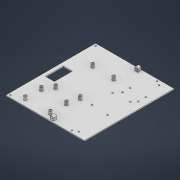
# Autodesk Inventor part: Obenplatte_vorne
Saved by Autodesk Inventor 2021 (Build 250183000, 183)
## iProperties
Created: 2021-02-01
Part Number: Obenplatte_vorne
Material: Generisch
Document SubType Name: Modeling
Designer: laure
Density: 1 g/cm^3
Appearance: Vorgabe
Author: laure
Autodesk Inventor part; units mm, degrees
ref_plane "YZ Plane" through (0, 0, 0) normal (1, 0, 0) x (0, 1, 0)
ref_plane "XZ Plane" through (0, 0, 0) normal (0, 1, 0) x (-1, 0, 0)
ref_plane "XY Plane" through (0, 0, 0) normal (0, 0, 1) x (1, 0, 0)
sketch "Skizze1" plane through (0, 0, 0) normal (0, 1, 0) x (-1, 0, 0)
  line L0 (87.5, -100) -> (-87.5, -100)
  line L1 (-87.5, -100) -> (-87.5, 100)
  line L2 (-87.5, 100) -> (87.5, 100)
  line L3 (87.5, 100) -> (87.5, -100)
  line L4 (0, -140) -> (0, 140) projected
  line L5 (122.5, 0) -> (-122.5, 0) projected
  point P0 (0, 0)
  dimension "d0" = 175
  dimension "d1" = 200
  constraints: 8 end point, 2 parallel, 1 horizontal, 1 perpendicular, 2 other
  measures "d0" distance of L1.end L2.end
  measures "d1" distance of L0.end L1.end
extrude "Extrusion1" add sketch "Skizze1" along normal blind 2
sketch "Skizze2" plane through (0, 2, 0) normal (0, 1, 0) x (1, 0, 0)
  circle A0 centre (54.5, 95) radius 1.6
  circle A1 centre (-82.5, 95) radius 1.6
  line L0 (0, 140) -> (0, -140) projected
  line L1 (122.5, 0) -> (-122.5, 0) projected
  line L2 (87.5, 100) -> (-87.5, 100) projected
  circle A2 centre (54.5, -95) radius 1.6
  circle A3 centre (-82.5, -95) radius 1.6
  line L3 (-87.5, 100) -> (-87.5, -100) projected
  line L4 (87.5, -100) -> (87.5, 100) projected
  point P0 (0, 0)
  dimension "d4" = 3.2
  dimension "d5" = 3.2
  dimension "d7" = 5
  dimension "d9" = 5
  dimension "d55" = 5
  dimension "d56" = 33
  constraints: 4 centre point, 2 symmetric about line, 2 other
  measures "d4" diameter of A0
  measures "d5" diameter of A1
  measures "d7" distance from line of L2 A0.centre
  measures "d9" distance from line of L2 A1.centre
  measures "d55" distance from line of L3 A1.centre
  measures "d56" distance from line of L4 A0.centre
extrude "Extrusion2" cut sketch "Skizze2" against normal up to surface (2 mm away) contours A0 | A1 | A2 | A3
sketch "Skizze3" plane through (0, 2, 0) normal (0, 1, 0) x (1, 0, 0)
  line L0 (0, 140) -> (0, -140) projected
  line L1 (122.5, 0) -> (-122.5, 0) projected
  line L2 (-87.5, -100) -> (87.5, -100) projected
  line L3 (-87.5, 100) -> (-87.5, -100) projected
  circle A0 centre (64.5, -89.5) radius 1.6
  line L4 (87.5, -100) -> (87.5, 100) projected
  circle A1 centre (64.5, -25.5) radius 1.6
  circle A2 centre (64.5, 25.5) radius 1.6
  line L5 (87.5, 100) -> (-87.5, 100) projected
  circle A3 centre (64.5, 89.5) radius 1.6
  circle A4 centre (27.5, -23) radius 1.6
  circle A5 centre (27.5, 23) radius 1.6
  point P0 (0, 0)
  dimension "d35" = 3.2
  dimension "d36" = 10.5
  dimension "d37" = 23
  dimension "d38" = 3.2
  dimension "d39" = 74.5
  dimension "d40" = 23
  dimension "d41" = 3.2
  dimension "d42" = 23
  dimension "d43" = 74.5
  dimension "d44" = 3.2
  dimension "d45" = 23
  dimension "d46" = 10.5
  dimension "d47" = 3.2
  dimension "d48" = 60
  dimension "d49" = 77
  dimension "d50" = 3.2
  dimension "d51" = 60
  dimension "d52" = 77
  constraints: 6 centre point
  measures "d35" diameter of A0
  measures "d36" distance from line of L2 A0.centre
  measures "d37" distance from line of L4 A0.centre
  measures "d38" diameter of A1
  measures "d39" distance from line of L2 A1.centre
  measures "d40" distance from line of L4 A1.centre
  measures "d41" diameter of A2
  measures "d42" distance from line of L4 A2.centre
  measures "d43" distance from line of L5 A2.centre
  measures "d44" diameter of A3
  measures "d45" distance from line of L4 A3.centre
  measures "d46" distance from line of L5 A3.centre
  measures "d47" diameter of A4
  measures "d48" distance from line of L4 A4.centre
  measures "d49" distance from line of L2 A4.centre
  measures "d50" diameter of A5
  measures "d51" distance from line of L4 A5.centre
  measures "d52" distance from line of L5 A5.centre
extrude "Extrusion3" cut sketch "Skizze3" against normal up to surface (2 mm away) contours A0 | A1 | A2 | A3 | A4 | A5
sketch "Skizze4" plane through (0, 2, 0) normal (0, 1, 0) x (1, 0, 0)
  line L0 (-47.5, -36.6) -> (5.84, -36.6)
  line L1 (5.84, -36.6) -> (5.84, 65)
  line L2 (5.84, 65) -> (-47.5, 65)
  line L3 (-47.5, 65) -> (-47.5, -36.6)
  line L4 (122.5, 0) -> (-122.5, 0) projected
  line L5 (-87.5, 100) -> (-87.5, -100) projected
  circle A0 centre (3.3, 49.76) radius 3.5
  circle A1 centre (3.3, -25.17) radius 3.5
  circle A2 centre (-44.96, -31.52) radius 3.5
  circle A3 centre (-44.96, 51.03) radius 3.5
  line L6 (87.5, 100) -> (-87.5, 100) projected
  point P0 (0, 0)
  point P1 (-15.83, 0)
  dimension "d57" = 53.34
  dimension "d58" = 101.6
  dimension "d59" = 40
  dimension "d60" = 7
  dimension "d61" = 86.36
  dimension "d62" = 50.8
  dimension "d63" = 7
  dimension "d64" = 90.17
  dimension "d65" = 50.8
  dimension "d66" = 7
  dimension "d67" = 96.52
  dimension "d68" = 50.8
  dimension "d69" = 7
  dimension "d70" = 87.63
  dimension "d71" = 50.8
  dimension "d140" = 35
  constraints: 8 end point, 4 centre point, 2 parallel, 1 horizontal, 1 perpendicular
  measures "d57" distance of L2.end L1.end
  measures "d58" distance of L1.end L0.end
  measures "d59" distance between parallel lines of L5 L3
  measures "d60" diameter of A0
  measures "d61" distance from line of L0 A0.centre
  measures "d62" distance from line of L3 A0.centre
  measures "d63" diameter of A1
  measures "d64" distance from line of L2 A1.centre
  measures "d65" distance from line of L3 A1.centre
  measures "d66" diameter of A2
  measures "d67" distance from line of L2 A2.centre
  measures "d68" distance from line of L1 A2.centre
  measures "d69" diameter of A3
  measures "d70" distance from line of L0 A3.centre
  measures "d71" distance from line of L1 A3.centre
  measures "d140" distance between parallel lines of L6 L2
extrude "Extrusion4" add sketch "Skizze4" along normal blind 7 contours A2 L3 | L3 A2 | A1 L1 | L1 A1 | A3 L3 | L3 A3 | A0 L1 | L1 A0
sketch "Skizze5" plane through (3.3, 9, -49.76) normal (0, 1, 0) x (1, 0, 0)
  circle A0 centre (0, 0) radius 3.5 projected
  circle A1 centre (-48.26, 1.27) radius 3.5 projected
  circle A2 centre (-48.26, -81.28) radius 3.5 projected
  circle A3 centre (0, -74.93) radius 3.5 projected
  circle A4 centre (0, 0) radius 2
  circle A5 centre (0, -74.93) radius 2
  circle A6 centre (-48.26, 1.27) radius 2
  circle A7 centre (-48.26, -81.28) radius 2
  point P0 (-3.3, -49.76)
  dimension "d74" = 4
  dimension "d75" = 4
  dimension "d76" = 4
  dimension "d77" = 4
  constraints: 4 centre point, 4 coincident
  measures "d74" diameter of A4
  measures "d75" diameter of A5
  measures "d76" diameter of A6
  measures "d77" diameter of A7
extrude "Extrusion5" cut sketch "Skizze5" against normal blind 5 contours A4 | A5 | A6 | A7
sketch "Skizze6" plane through (0, 2, 0) normal (0, 1, 0) x (1, 0, 0)
  circle A0 centre (72.5, 35) radius 1.6
  circle A1 centre (72.5, 52) radius 1.6
  line L0 (87.5, -100) -> (87.5, 100) projected
  line L1 (-122.5, 0) -> (122.5, 0) projected
  circle A2 centre (37.5, 35) radius 1.6
  circle A3 centre (37.5, 52) radius 1.6
  point P0 (0, 0)
  dimension "d80" = 3.2
  dimension "d81" = 3.2
  dimension "d82" = 15
  dimension "d83" = 15
  dimension "d84" = 35
  dimension "d85" = 17
  dimension "d88" = 3.2
  dimension "d89" = 3.2
  dimension "d90" = 50
  dimension "d91" = 50
  dimension "d92" = 35
  dimension "d94" = 17
  constraints: 4 centre point
  measures "d80" diameter of A0
  measures "d81" diameter of A1
  measures "d82" distance from line of L0 A0.centre
  measures "d83" distance from line of L0 A1.centre
  measures "d84" distance from line of L1 A0.centre
  measures "d85" distance of A0.centre A1.centre
  measures "d88" diameter of A2
  measures "d89" diameter of A3
  measures "d90" distance from line of L0 A2.centre
  measures "d91" distance from line of L0 A3.centre
  measures "d92" distance from line of L1 A2.centre
  measures "d94" distance of A2.centre A3.centre
extrude "Extrusion6" cut sketch "Skizze6" against normal up to surface (2 mm away)
sketch "Skizze7" plane through (0, 2, 0) normal (0, 1, 0) x (1, 0, 0)
  line L0 (16, -90.8) -> (9, -90.8)
  line L1 (9, -90.8) -> (9, -97.8)
  line L2 (9, -97.8) -> (16, -97.8)
  line L3 (16, -97.8) -> (16, -90.8)
  line L4 (-87.5, 100) -> (-87.5, -100) projected
  line L5 (-87.5, -100) -> (87.5, -100) projected
  line L6 (122.5, 0) -> (-122.5, 0) projected
  line L7 (16, 90.8) -> (9, 90.8)
  line L8 (9, 90.8) -> (9, 97.8)
  line L9 (9, 97.8) -> (16, 97.8)
  line L10 (16, 97.8) -> (16, 90.8)
  point P0 (0, 0)
  dimension "d95" = 103.5
  dimension "d96" = 7
  dimension "d97" = 7
  dimension "d98" = 2.2
  constraints: 16 end point, 4 symmetric about line, 2 parallel, 1 horizontal, 1 perpendicular
  measures "d95" distance between parallel lines of L4 L3
  measures "d96" distance between parallel lines of L3 L1
  measures "d97" distance between parallel lines of L2 L0
  measures "d98" distance between parallel lines of L5 L2
extrude "Extrusion7" add sketch "Skizze7" along normal blind 9
sketch "Skizze8" plane through (9, 2, 97.8) normal (0, 0, 1) x (1, 0, 0)
  circle A0 centre (3.5, 5) radius 2
  line L0 (7, 0) -> (0, 0) projected
  line L1 (7, 0) -> (7, 9) projected
  point P0 (-9, -2)
  dimension "d101" = 4
  dimension "d102" = 5
  dimension "d103" = 3.5
  constraints: 1 centre point
  measures "d101" diameter of A0
  measures "d102" distance from line of L0 A0.centre
  measures "d103" distance from line of L1 A0.centre
extrude "Extrusion8" cut sketch "Skizze8" against normal blind 5
sketch "Skizze9" plane through (16, 2, -97.8) normal (0, 0, -1) x (-1, 0, 0)
  circle A0 centre (3.5, 5) radius 2
  line L0 (7, 0) -> (7, 9) projected
  line L1 (7, 0) -> (0, 0) projected
  point P0 (16, -2)
  dimension "d107" = 4
  dimension "d108" = 3.5
  dimension "d109" = 5
  constraints: 1 centre point
  measures "d107" diameter of A0
  measures "d108" distance from line of L0 A0.centre
  measures "d109" distance from line of L1 A0.centre
extrude "Extrusion9" cut sketch "Skizze9" against normal blind 5
fillet "Rundung1" radius 3.5 4 edges at (16, 11, -94.3) (9, 11, -94.3) (9, 11, 94.3) (16, 11, 94.3)
sketch "Skizze10" plane through (0, 2, 0) normal (0, 1, 0) x (1, 0, 0)
  line L0 (-59.5, 20) -> (-79.5, 20)
  line L1 (-79.5, 20) -> (-79.5, -20)
  line L2 (-79.5, -20) -> (-59.5, -20)
  line L3 (-59.5, -20) -> (-59.5, 20)
  line L4 (122.5, 0) -> (-122.5, 0) projected
  line L5 (-87.5, 100) -> (-87.5, -100) projected
  point P0 (0, 0)
  dimension "d113" = 20
  dimension "d114" = 40
  dimension "d115" = 8
  constraints: 8 end point, 2 parallel, 1 horizontal, 1 perpendicular, 1 other
  measures "d113" distance of L2.end L1.end
  measures "d114" distance of L1.end L0.end
  measures "d115" distance between parallel lines of L5 L1
extrude "Extrusion10" cut sketch "Skizze10" against normal up to surface (2 mm away)
sketch "Skizze11" plane through (0, 2, 0) normal (0, 1, 0) x (1, 0, 0)
  circle A0 centre (-1.5, -51) radius 3.5
  circle A1 centre (-1.5, -87) radius 3.5
  circle A2 centre (-57.5, -51) radius 3.5
  circle A3 centre (-57.5, -87) radius 3.5
  line L0 (-87.5, 100) -> (-87.5, -100) projected
  line L1 (87.5, 100) -> (-87.5, 100) projected
  line L2 (-87.5, -100) -> (87.5, -100) projected
  point P0 (0, 0)
  dimension "d118" = 7
  dimension "d119" = 7
  dimension "d120" = 7
  dimension "d121" = 7
  dimension "d122" = 30
  dimension "d123" = 30
  dimension "d126" = 56
  dimension "d127" = 36
  dimension "d128" = 56
  dimension "d129" = 36
  dimension "d138" = 13
  dimension "d139" = 13
  constraints: 4 centre point
  measures "d118" diameter of A0
  measures "d119" diameter of A1
  measures "d120" diameter of A2
  measures "d121" diameter of A3
  measures "d122" distance from line of A2.centre L0
  measures "d123" distance from line of L0 A3.centre
  measures "d126" distance of A2.centre A0.centre
  measures "d127" distance of A2.centre A3.centre
  measures "d128" distance of A3.centre A1.centre
  measures "d129" distance of A0.centre A1.centre
  measures "d138" distance from line of L2 A1.centre
  measures "d139" distance from line of L2 A3.centre
extrude "Extrusion11" add sketch "Skizze11" along normal blind 7
sketch "Skizze12" plane through (-1.5, 9, 51) normal (0, 1, 0) x (1, 0, 0)
  circle A0 centre (0, 0) radius 3.5 projected
  circle A1 centre (0, -36) radius 3.5 projected
  circle A2 centre (-56, -36) radius 3.5 projected
  circle A3 centre (-56, 0) radius 3.5 projected
  circle A4 centre (0, 0) radius 2.15
  circle A5 centre (0, -36) radius 2.15
  circle A6 centre (-56, 0) radius 2.15
  circle A7 centre (-56, -36) radius 2.15
  point P0 (1.5, 51)
  dimension "d132" = 4.3
  dimension "d133" = 4.3
  dimension "d134" = 4.3
  dimension "d135" = 4.3
  constraints: 4 centre point, 4 coincident
  measures "d132" diameter of A4
  measures "d133" diameter of A5
  measures "d134" diameter of A6
  measures "d135" diameter of A7
extrude "Extrusion12" cut sketch "Skizze12" against normal blind 6 contours A4 | A5 | A6 | A7
equation "\"d10\" = d6"
equation "\"d53\" = d48"
equation "\"d6\" = 42"
